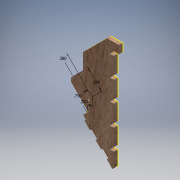
# Autodesk Inventor part: MarkerShaftBot
Saved by Autodesk Inventor 2019 (Build 230136000, 136)
## iProperties
Created: 2019-01-14
Part Number: MarkerShaftBot
Material: Wood (Birch)
Document SubType Name: Modeling
Designer: nxgam
Density: 0.55 g/cm^3
Appearance: Birch - Natural Polished
Mass: 12.9015 g
Surface Area: 113.899 cm^2
Volume: 23.4572 cm^3
Author: nxgam
Autodesk Inventor part; units mm, degrees
ref_plane "YZ Plane" through (0, 0, 0) normal (1, 0, 0) x (0, 1, 0)
ref_plane "XZ Plane" through (0, 0, 0) normal (0, 1, 0) x (-1, 0, 0)
ref_plane "XY Plane" through (0, 0, 0) normal (0, 0, 1) x (1, 0, 0)
sketch "Sketch1" plane through (0, 0, 0) normal (0, 0, 1) x (1, 0, 0)
  line L0 (0, 0) -> (10.16, 0)
  line L1 (10.16, 0) -> (10.16, 132.08)
  line L2 (10.16, 132.08) -> (0, 132.08)
  line L3 (0, 132.08) -> (0, 0)
  line L4 (10.16, 10.16) -> (5.08, 10.16)
  line L5 (5.08, 10.16) -> (5.08, 15.24)
  line L6 (5.08, 15.24) -> (10.16, 15.24)
  line L7 (10.16, 15.24) -> (10.16, 10.16)
  line L8 (10.16, 36.83) -> (5.08, 36.83)
  line L9 (5.08, 36.83) -> (5.08, 41.91)
  line L10 (5.08, 41.91) -> (10.16, 41.91)
  line L11 (10.16, 41.91) -> (10.16, 36.83)
  line L12 (10.16, 63.5) -> (5.08, 63.5)
  line L13 (5.08, 63.5) -> (5.08, 68.58)
  line L14 (5.08, 68.58) -> (10.16, 68.58)
  line L15 (10.16, 68.58) -> (10.16, 63.5)
  line L16 (10.16, 90.17) -> (5.08, 90.17)
  line L17 (5.08, 90.17) -> (5.08, 95.25)
  line L18 (5.08, 95.25) -> (10.16, 95.25)
  line L19 (10.16, 95.25) -> (10.16, 90.17)
  line L20 (10.16, 116.84) -> (5.08, 116.84)
  line L21 (5.08, 116.84) -> (5.08, 121.92)
  line L22 (5.08, 121.92) -> (10.16, 121.92)
  line L23 (10.16, 121.92) -> (10.16, 116.84)
  dimension "d0" = 10.16
  dimension "d1" = 132.08
  dimension "d2" = 5.08
  dimension "d3" = 5.08
  dimension "d4" = 10.16
  dimension "d7" = 26.67
  constraints: 48 end point, 4 parallel, 2 horizontal, 2 perpendicular, 1 point on line, 1 vertical, 32 other
  measures "d0" distance of L2.end L1.end
  measures "d1" distance of L1.end L0.end
  measures "d2" distance of L5.end L6.end
  measures "d3" distance of L4.end L5.end
  measures "d4" distance between parallel lines of L0 L4
  measures "d7" distance of L4.start L8.start
extrude "Extrusion2" add sketch "Sketch1" along normal blind 5.08 contours L3 L2 L1 L22 L21 L20 L18 L17 L16 L14 L13 L12 L10 L9 L8 L6 L5 L4 L0
thicken "Thicken3" operation add thickness 5.08 both sides no extend neighbours yes toward (-1, 0, 0) faces at (0, 88.0533, 1.6933)
thicken "Thicken4" operation add thickness 6.35 both sides no extend neighbours yes toward (1, 0, 0) faces at (10.16, 125.3067, 3.3867)
chamfer "Chamfer2" distance 6.35 angle 45 1 edges at (-5.08, 132.08, 2.54)
sketch "Sketch2" plane through (0, 0, 5.08) normal (0, 0, 1) x (1, 0, 0)
  line L0 (-5.08, 125.73) -> (1.27, 132.08) projected
  line L1 (-5.08, 125.73) -> (-5.08, 0) projected
  line L2 (-5.08, 0) -> (10.16, 0) projected
  line L3 (10.16, 0) -> (10.16, 10.16) projected
  line L4 (10.16, 10.16) -> (5.08, 10.16) projected
  line L5 (5.08, 10.16) -> (5.08, 15.24) projected
  line L6 (5.08, 15.24) -> (10.16, 15.24) projected
  line L7 (10.16, 15.24) -> (10.16, 36.83) projected
  line L8 (10.16, 36.83) -> (5.08, 36.83) projected
  line L9 (5.08, 36.83) -> (5.08, 41.91) projected
  line L10 (5.08, 41.91) -> (10.16, 41.91) projected
  line L11 (10.16, 41.91) -> (10.16, 63.5) projected
  line L12 (10.16, 63.5) -> (5.08, 63.5) projected
  line L13 (5.08, 63.5) -> (5.08, 68.58) projected
  line L14 (5.08, 68.58) -> (10.16, 68.58) projected
  line L15 (10.16, 68.58) -> (10.16, 90.17) projected
  line L16 (10.16, 90.17) -> (5.08, 90.17) projected
  line L17 (5.08, 90.17) -> (5.08, 95.25) projected
  line L18 (5.08, 95.25) -> (10.16, 95.25) projected
  line L19 (10.16, 95.25) -> (10.16, 116.84) projected
  line L20 (10.16, 116.84) -> (5.08, 116.84) projected
  line L21 (5.08, 116.84) -> (5.08, 121.92) projected
  line L22 (5.08, 121.92) -> (16.51, 121.92) projected
  line L23 (16.51, 121.92) -> (16.51, 132.08) projected
  line L24 (16.51, 132.08) -> (1.27, 132.08) projected
  line L25 (-5.08, 125.73) -> (-67.945, 62.865)
  line L26 (-5.08, 0) -> (10.16, 0) projected
  line L27 (-67.945, 62.865) -> (-5.08, 0)
  line L28 (-5.08, 0) -> (10.16, -15.24)
  line L29 (10.16, -15.24) -> (10.16, 0)
  line L30 (-5.08, 125.73) -> (1.27, 132.08) projected
  line L31 (10.16, 0) -> (10.16, 10.16) projected
  point P0 (0, 0)
  constraints: 8 end point, 2 collinear, 2 perpendicular
extrude "Extrusion3" add sketch "Sketch2" against normal blind 5.08 contours L1 L27 L25 | L2 L29 L28
sketch "Sketch3" plane through (0, 0, 5.08) normal (0, 0, 1) x (1, 0, 0)
  line L0 (1.27, 132.08) -> (-67.945, 62.865) projected
  line L1 (-67.945, 62.865) -> (10.16, -15.24) projected
  line L2 (10.16, -15.24) -> (10.16, 10.16) projected
  line L3 (10.16, 10.16) -> (5.08, 10.16) projected
  line L4 (5.08, 10.16) -> (5.08, 15.24) projected
  line L5 (5.08, 15.24) -> (10.16, 15.24) projected
  line L6 (10.16, 15.24) -> (10.16, 36.83) projected
  line L7 (10.16, 36.83) -> (5.08, 36.83) projected
  line L8 (5.08, 36.83) -> (5.08, 41.91) projected
  line L9 (5.08, 41.91) -> (10.16, 41.91) projected
  line L10 (10.16, 41.91) -> (10.16, 63.5) projected
  line L11 (10.16, 63.5) -> (5.08, 63.5) projected
  line L12 (5.08, 63.5) -> (5.08, 68.58) projected
  line L13 (5.08, 68.58) -> (10.16, 68.58) projected
  line L14 (10.16, 68.58) -> (10.16, 90.17) projected
  line L15 (10.16, 90.17) -> (5.08, 90.17) projected
  line L16 (5.08, 90.17) -> (5.08, 95.25) projected
  line L17 (5.08, 95.25) -> (10.16, 95.25) projected
  line L18 (10.16, 95.25) -> (10.16, 116.84) projected
  line L19 (10.16, 116.84) -> (5.08, 116.84) projected
  line L20 (5.08, 116.84) -> (5.08, 121.92) projected
  line L21 (5.08, 121.92) -> (16.51, 121.92) projected
  line L22 (16.51, 121.92) -> (16.51, 132.08) projected
  line L23 (16.51, 132.08) -> (1.27, 132.08) projected
  line L24 (10.16, -15.24) -> (10.16, 10.16) projected
  line L25 (10.16, -8.0558) -> (-64.3529, 66.4571)
  line L26 (-67.945, 62.865) -> (10.16, -15.24) projected
  line L27 (-64.3529, 66.4571) -> (-67.945, 62.865)
  line L28 (10.16, -8.0558) -> (10.16, -15.24)
  line L29 (-67.945, 62.865) -> (10.16, -15.24)
  point P0 (0, 0)
  dimension "d32" = 5.08
  constraints: 8 end point, 2 collinear, 2 point on line, 1 parallel
  measures "d32" distance between parallel lines of L26 L25
extrude "Extrusion4" cut sketch "Sketch3" against normal blind 5.08 contours L25 L2 L1 L0
sketch "Sketch4" plane through (0, 0, 5.08) normal (0, 0, 1) x (1, 0, 0)
  line L0 (37.592, 132.08) -> (53.2638, 116.4082) projected
  line L1 (22.352, 132.08) -> (37.592, 132.08) projected
  line L2 (22.352, 121.92) -> (22.352, 132.08) projected
  line L3 (22.352, 121.92) -> (33.782, 121.92) projected
  line L4 (33.782, 121.92) -> (33.782, 116.84) projected
  line L5 (33.782, 116.84) -> (28.702, 116.84) projected
  line L6 (28.702, 95.25) -> (28.702, 116.84) projected
  line L7 (28.702, 95.25) -> (33.782, 95.25) projected
  line L8 (33.782, 95.25) -> (33.782, 90.17) projected
  line L9 (33.782, 90.17) -> (28.702, 90.17) projected
  line L10 (28.702, 68.58) -> (28.702, 90.17) projected
  line L11 (28.702, 68.58) -> (33.782, 68.58) projected
  line L12 (33.782, 68.58) -> (33.782, 63.5) projected
  line L13 (33.782, 63.5) -> (28.702, 63.5) projected
  line L14 (28.702, 41.91) -> (28.702, 63.5) projected
  line L15 (28.702, 41.91) -> (33.782, 41.91) projected
  line L16 (33.782, 41.91) -> (33.782, 36.83) projected
  line L17 (33.782, 36.83) -> (28.702, 36.83) projected
  line L18 (28.702, 15.24) -> (28.702, 36.83) projected
  line L19 (28.702, 15.24) -> (33.782, 15.24) projected
  line L20 (33.782, 15.24) -> (33.782, 10.16) projected
  line L21 (33.782, 10.16) -> (28.702, 10.16) projected
  line L22 (28.702, 10.16) -> (28.702, -26.5978) projected
  line L23 (28.702, -26.5978) -> (31.7112, -29.607) projected
  line L24 (29.7355, -31.5826) -> (31.7112, -29.607) projected
  line L25 (36.9197, -38.7668) -> (29.7355, -31.5826) projected
  line L26 (38.8954, -36.7912) -> (36.9197, -38.7668) projected
  line L27 (38.8954, -36.7912) -> (46.0796, -43.9754) projected
  line L28 (46.0796, -43.9754) -> (44.1039, -45.951) projected
  line L29 (44.1039, -45.951) -> (51.2881, -53.1353) projected
  line L30 (53.2638, -10.5688) -> (53.2638, 116.4082) projected
  line L31 (36.9197, -38.7668) -> (29.7355, -31.5826)
  line L32 (29.7355, -31.5826) -> (31.7112, -29.607)
  line L33 (31.7112, -29.607) -> (38.8954, -36.7912)
  line L34 (38.8954, -36.7912) -> (36.9197, -38.7668)
  line L35 (15.3671, -17.2142) -> (17.3428, -15.2386)
  line L36 (17.3428, -15.2386) -> (24.527, -22.4228)
  line L37 (22.5513, -24.3984) -> (15.3671, -17.2142)
  line L38 (24.527, -22.4228) -> (22.5513, -24.3984)
  line L39 (0.9987, -2.8458) -> (2.9744, -0.8702)
  line L40 (2.9744, -0.8702) -> (10.1586, -8.0544)
  line L41 (8.1829, -10.03) -> (0.9987, -2.8458)
  line L42 (10.1586, -8.0544) -> (8.1829, -10.03)
  line L43 (-13.3697, 11.5226) -> (-11.394, 13.4982)
  line L44 (-11.394, 13.4982) -> (-4.2098, 6.314)
  line L45 (-6.1855, 4.3384) -> (-13.3697, 11.5226)
  line L46 (-4.2098, 6.314) -> (-6.1855, 4.3384)
  line L47 (-27.7381, 25.891) -> (-25.7625, 27.8667)
  line L48 (-25.7625, 27.8667) -> (-18.5782, 20.6825)
  line L49 (-20.5539, 18.7068) -> (-27.7381, 25.891)
  line L50 (-18.5782, 20.6825) -> (-20.5539, 18.7068)
  line L51 (-42.1065, 40.2594) -> (-40.1309, 42.2351)
  line L52 (-40.1309, 42.2351) -> (-32.9467, 35.0509)
  line L53 (-34.9223, 33.0752) -> (-42.1065, 40.2594)
  line L54 (-32.9467, 35.0509) -> (-34.9223, 33.0752)
  line L55 (-56.4749, 54.6278) -> (-54.4993, 56.6035)
  line L56 (-54.4993, 56.6035) -> (-47.3151, 49.4193)
  line L57 (-49.2907, 47.4436) -> (-56.4749, 54.6278)
  line L58 (-47.3151, 49.4193) -> (-49.2907, 47.4436)
  line L59 (-70.8433, 68.9962) -> (-68.8677, 70.9719)
  line L60 (-68.8677, 70.9719) -> (-61.6835, 63.7877)
  line L61 (-63.6591, 61.812) -> (-70.8433, 68.9962)
  line L62 (-61.6835, 63.7877) -> (-63.6591, 61.812)
  circle A0 centre (49.1329, -20.0879) radius 2 projected
  line L63 (51.2881, -53.1353) -> (71.3141, -33.1093) projected
  line L64 (71.3141, -28.6192) -> (53.2638, -10.5688) projected
  line L65 (71.3141, -28.6192) -> (71.3141, -33.1093) projected
  point P0 (0, 0)
  point P1 (53.2638, -51.1596)
  dimension "d35" = 2.794
  dimension "d38" = 20.32
  constraints: 64 end point, 3 equal length, 1 perpendicular, 57 other
  measures "d35" distance between parallel lines of L25 L33
  measures "d38" distance of L32.end L35.end
extrude "Extrusion5" add sketch "Sketch4" against normal blind 5.08 contours L39 L40 L42 L41 | L43 L44 L46 L45 | L47 L48 L50 L49 | L51 L52 L54 L53 | L55 L56 L58 L57
sketch "Sketch5" plane through (0, 0, 0) normal (0, 0, -1) x (-1, 0, 0)
  line L0 (-10.16, -8.0558) -> (-10.1586, -8.0544) projected
  line L1 (-10.1586, -8.0544) -> (-8.1829, -10.03) projected
  line L2 (-8.1829, -10.03) -> (-0.9987, -2.8458) projected
  line L3 (-0.9987, -2.8458) -> (-2.9744, -0.8702) projected
  line L4 (-2.9744, -0.8702) -> (4.2098, 6.314) projected
  line L5 (4.2098, 6.314) -> (6.1855, 4.3384) projected
  line L6 (6.1855, 4.3384) -> (13.3697, 11.5226) projected
  line L7 (13.3697, 11.5226) -> (11.394, 13.4982) projected
  line L8 (11.394, 13.4982) -> (18.5782, 20.6825) projected
  line L9 (18.5782, 20.6825) -> (20.5539, 18.7068) projected
  line L10 (20.5539, 18.7068) -> (27.7381, 25.891) projected
  line L11 (27.7381, 25.891) -> (25.7625, 27.8667) projected
  line L12 (25.7625, 27.8667) -> (32.9467, 35.0509) projected
  line L13 (32.9467, 35.0509) -> (34.9223, 33.0752) projected
  line L14 (34.9223, 33.0752) -> (42.1065, 40.2594) projected
  line L15 (42.1065, 40.2594) -> (40.1309, 42.2351) projected
  line L16 (40.1309, 42.2351) -> (47.3151, 49.4193) projected
  line L17 (47.3151, 49.4193) -> (49.2907, 47.4436) projected
  line L18 (49.2907, 47.4436) -> (56.4749, 54.6278) projected
  line L19 (56.4749, 54.6278) -> (54.4993, 56.6035) projected
  line L20 (54.4993, 56.6035) -> (64.3529, 66.4571) projected
  line L21 (-1.27, 132.08) -> (64.3529, 66.4571) projected
  line L22 (-16.51, 132.08) -> (-1.27, 132.08) projected
  line L23 (-16.51, 121.92) -> (-16.51, 132.08) projected
  line L24 (-16.51, 121.92) -> (-5.08, 121.92) projected
  line L25 (-5.08, 121.92) -> (-5.08, 116.84) projected
  line L26 (-5.08, 116.84) -> (-10.16, 116.84) projected
  line L27 (-10.16, 95.25) -> (-10.16, 116.84) projected
  line L28 (-10.16, 95.25) -> (-5.08, 95.25) projected
  line L29 (-5.08, 95.25) -> (-5.08, 90.17) projected
  line L30 (-5.08, 90.17) -> (-10.16, 90.17) projected
  line L31 (-10.16, 68.58) -> (-10.16, 90.17) projected
  line L32 (-10.16, 68.58) -> (-5.08, 68.58) projected
  line L33 (-5.08, 68.58) -> (-5.08, 63.5) projected
  line L34 (-5.08, 63.5) -> (-10.16, 63.5) projected
  line L35 (-10.16, 41.91) -> (-10.16, 63.5) projected
  line L36 (-10.16, 41.91) -> (-5.08, 41.91) projected
  line L37 (-5.08, 41.91) -> (-5.08, 36.83) projected
  line L38 (-5.08, 36.83) -> (-10.16, 36.83) projected
  line L39 (-10.16, 15.24) -> (-10.16, 36.83) projected
  line L40 (-10.16, 15.24) -> (-5.08, 15.24) projected
  line L41 (-5.08, 15.24) -> (-5.08, 10.16) projected
  line L42 (-5.08, 10.16) -> (-10.16, 10.16) projected
  line L43 (-10.16, 10.16) -> (-10.16, -8.0558) projected
  line L44 (29.3546, 31.4588) -> (29.3546, 109.6224)
  line L45 (29.3546, 109.6224) -> (97.3324, 52.705)
  line L46 (97.3324, 52.705) -> (38.3891, 15.24)
  line L47 (38.3891, 15.24) -> (29.3546, 31.4588)
  point P0 (0, 0)
  constraints: 8 end point, 1 midpoint, 1 vertical
extrude "Extrusion6" cut sketch "Sketch5" against normal blind 5.08 contours L44 L21 L20 L19 L18 L17 L16 L15 L14 L13 L12 | L12 L13 L14 L15 L16 L17 L18 L19 L20 L21 L44 L45 L46 L47
sketch "Sketch6" plane through (0, 0, 0) normal (0, 0, -1) x (-1, 0, 0)
  line L0 (29.3546, 31.4588) -> (29.3546, 101.4554) projected
  line L1 (-1.27, 132.08) -> (29.3546, 101.4554) projected
  line L2 (-16.51, 132.08) -> (-1.27, 132.08) projected
  line L3 (-16.51, 121.92) -> (-16.51, 132.08) projected
  line L4 (-16.51, 121.92) -> (-5.08, 121.92) projected
  line L5 (-5.08, 121.92) -> (-5.08, 116.84) projected
  line L6 (-5.08, 116.84) -> (-10.16, 116.84) projected
  line L7 (-10.16, 95.25) -> (-10.16, 116.84) projected
  line L8 (-10.16, 95.25) -> (-5.08, 95.25) projected
  line L9 (-5.08, 95.25) -> (-5.08, 90.17) projected
  line L10 (-5.08, 90.17) -> (-10.16, 90.17) projected
  line L11 (-10.16, 68.58) -> (-10.16, 90.17) projected
  line L12 (-10.16, 68.58) -> (-5.08, 68.58) projected
  line L13 (-5.08, 68.58) -> (-5.08, 63.5) projected
  line L14 (-5.08, 63.5) -> (-10.16, 63.5) projected
  line L15 (-10.16, 41.91) -> (-10.16, 63.5) projected
  line L16 (-10.16, 41.91) -> (-5.08, 41.91) projected
  line L17 (-5.08, 41.91) -> (-5.08, 36.83) projected
  line L18 (-5.08, 36.83) -> (-10.16, 36.83) projected
  line L19 (-10.16, 15.24) -> (-10.16, 36.83) projected
  line L20 (-10.16, 15.24) -> (-5.08, 15.24) projected
  line L21 (-5.08, 15.24) -> (-5.08, 10.16) projected
  line L22 (-5.08, 10.16) -> (-10.16, 10.16) projected
  line L23 (-10.16, 10.16) -> (-10.16, -8.0558) projected
  line L24 (-10.16, -8.0558) -> (-10.1586, -8.0544) projected
  line L25 (-10.1586, -8.0544) -> (-8.1829, -10.03) projected
  line L26 (-8.1829, -10.03) -> (-0.9987, -2.8458) projected
  line L27 (-0.9987, -2.8458) -> (-2.9744, -0.8702) projected
  line L28 (-2.9744, -0.8702) -> (4.2098, 6.314) projected
  line L29 (4.2098, 6.314) -> (6.1855, 4.3384) projected
  line L30 (6.1855, 4.3384) -> (13.3697, 11.5226) projected
  line L31 (13.3697, 11.5226) -> (11.394, 13.4982) projected
  line L32 (11.394, 13.4982) -> (18.5782, 20.6825) projected
  line L33 (18.5782, 20.6825) -> (20.5539, 18.7068) projected
  line L34 (20.5539, 18.7068) -> (27.7381, 25.891) projected
  line L35 (27.7381, 25.891) -> (25.7625, 27.8667) projected
  line L36 (25.7625, 27.8667) -> (29.3546, 31.4588) projected
  line L37 (29.3546, 101.4554) -> (29.3546, 31.4588) projected
  line L38 (29.3546, 80.9021) -> (47.4309, 62.8258)
  line L39 (47.4309, 62.8258) -> (29.3546, 44.7495)
  line L40 (29.3546, 44.7495) -> (29.3546, 80.9021)
  line L41 (29.3546, 31.4588) -> (29.3546, 101.4554) projected
  line L42 (27.7381, 25.891) -> (25.7625, 27.8667) projected
  point P0 (0, 0)
  point P1 (23.0046, 52.0495)
  dimension "d47" = 24.892
  dimension "d48" = 9.652
  dimension "d49" = 19.05
  dimension "d59" = 6.35
  constraints: 6 end point, 2 point on line, 1 parallel, 1 perpendicular
  measures "d47" distance from line of L38 point (23.005, 52.05)
  measures "d48" distance from line of L39 point (23.005, 52.05)
  measures "d49" distance from line of L36 point (23.005, 52.05)
  measures "d59" horizontal distance of point (23.005, 52.05) L0.start
extrude "Extrusion7" add sketch "Sketch6" against normal blind 5.08 contours L0 L38 L39
hole "Hole1" at (-23.0046, 52.0495, 0) direction (0, 0, 1) diameter 4 end through all
chamfer "Chamfer3" distance 3.175 angle 45 1 edges at (-47.4309, 62.8258, 2.54)
sketch "Sketch7" plane through (0, 0, 0) normal (0, 0, -1) x (-1, 0, 0)
  line L0 (45.1858, 65.0709) -> (45.1858, 60.5808) projected
  line L1 (45.1858, 65.0709) -> (29.3546, 80.9021) projected
  line L2 (29.3546, 80.9021) -> (29.3546, 101.4554) projected
  line L3 (-1.27, 132.08) -> (29.3546, 101.4554) projected
  line L4 (-16.51, 132.08) -> (-1.27, 132.08) projected
  line L5 (-16.51, 121.92) -> (-16.51, 132.08) projected
  line L6 (-16.51, 121.92) -> (-5.08, 121.92) projected
  line L7 (-5.08, 121.92) -> (-5.08, 116.84) projected
  line L8 (-5.08, 116.84) -> (-10.16, 116.84) projected
  line L9 (-10.16, 95.25) -> (-10.16, 116.84) projected
  line L10 (-10.16, 95.25) -> (-5.08, 95.25) projected
  line L11 (-5.08, 95.25) -> (-5.08, 90.17) projected
  line L12 (-5.08, 90.17) -> (-10.16, 90.17) projected
  line L13 (-10.16, 68.58) -> (-10.16, 90.17) projected
  line L14 (-10.16, 68.58) -> (-5.08, 68.58) projected
  line L15 (-5.08, 68.58) -> (-5.08, 63.5) projected
  line L16 (-5.08, 63.5) -> (-10.16, 63.5) projected
  line L17 (-10.16, 41.91) -> (-10.16, 63.5) projected
  line L18 (-10.16, 41.91) -> (-5.08, 41.91) projected
  line L19 (-5.08, 41.91) -> (-5.08, 36.83) projected
  line L20 (-5.08, 36.83) -> (-10.16, 36.83) projected
  line L21 (-10.16, 15.24) -> (-10.16, 36.83) projected
  line L22 (-10.16, 15.24) -> (-5.08, 15.24) projected
  line L23 (-5.08, 15.24) -> (-5.08, 10.16) projected
  line L24 (-5.08, 10.16) -> (-10.16, 10.16) projected
  line L25 (-10.16, 10.16) -> (-10.16, -8.0558) projected
  line L26 (-10.16, -8.0558) -> (-10.1586, -8.0544) projected
  line L27 (-10.1586, -8.0544) -> (-8.1829, -10.03) projected
  line L28 (-8.1829, -10.03) -> (-0.9987, -2.8458) projected
  line L29 (-0.9987, -2.8458) -> (-2.9744, -0.8702) projected
  line L30 (-2.9744, -0.8702) -> (4.2098, 6.314) projected
  line L31 (4.2098, 6.314) -> (6.1855, 4.3384) projected
  line L32 (6.1855, 4.3384) -> (13.3697, 11.5226) projected
  line L33 (13.3697, 11.5226) -> (11.394, 13.4982) projected
  line L34 (11.394, 13.4982) -> (18.5782, 20.6825) projected
  line L35 (18.5782, 20.6825) -> (20.5539, 18.7068) projected
  line L36 (20.5539, 18.7068) -> (27.7381, 25.891) projected
  line L37 (27.7381, 25.891) -> (25.7625, 27.8667) projected
  line L38 (25.7625, 27.8667) -> (29.3546, 31.4588) projected
  line L39 (29.3546, 31.4588) -> (29.3546, 44.7495) projected
  line L40 (29.3546, 44.7495) -> (45.1858, 60.5808) projected
  circle A0 centre (23.0046, 52.0495) radius 2 projected
  line L41 (29.3546, 31.4588) -> (22.7092, 38.1042)
  line L42 (22.7092, 38.1042) -> (29.3546, 44.7495)
  line L43 (29.3546, 44.7495) -> (29.3546, 31.4588) projected
  line L44 (29.3546, 31.4588) -> (29.3546, 44.7495)
  line L45 (29.3546, 44.7495) -> (45.1858, 60.5808) projected
  point P0 (0, 0)
  constraints: 6 end point, 1 collinear, 1 perpendicular, 1 vertical
extrude "Extrusion8" cut sketch "Sketch7" against normal blind 5.08 contours L39 L41 L42
body "Solid2"
